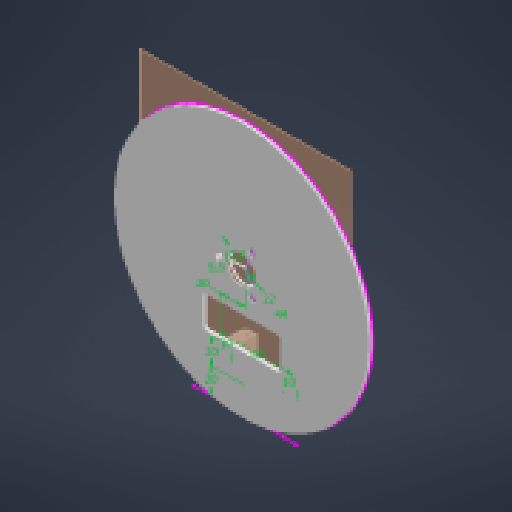
# Autodesk Inventor part: Pokrywa_góra
Saved by Autodesk Inventor 2025 (Build 290162000, 162)
## iProperties
Created: 2024-04-14
Part Number: Pokrywa_góra
Material: Generic
Document SubType Name: Modeling
Designer: sicia
Density: 1 g/cm^3
Appearance: Default
Author: sicia
Autodesk Inventor part; units mm, degrees
ref_plane "YZ Plane" through (0, 0, 0) normal (1, 0, 0) x (0, 1, 0)
ref_plane "XZ Plane" through (0, 0, 0) normal (0, 1, 0) x (-1, 0, 0)
ref_plane "XY Plane" through (0, 0, 0) normal (0, 0, 1) x (1, 0, 0)
ref_plane "Work Plane1" through (0, 0, 0) normal (0, 0, 1) x (1, 0, 0)
ref_plane "Work Plane2" through (0, 0, 0) normal (0, 0, 1) x (1, 0, 0)
sketch "Sketch3" plane through (0, 0, 0) normal (0, 0, 1) x (1, 0, 0)
  circle A0 centre (-75, -25) radius 100 projected
  circle A1 centre (-75, -25) radius 95 projected
  point P0 (-75, -25)
  point P1 (-75, -25)
  point P2 (-75, -25)
  point P3 (-75, -25)
extrude "Extrusion3" add sketch "Sketch3" along normal blind 3 contours A0 | A1
sketch "Sketch9" plane through (0, 0, 0) normal (0, 0, -1) x (-1, 0, 0)
  line L0 (115, -125) -> (35, -125) projected
  line L1 (35, -105) -> (95, -105)
  line L2 (95, -105) -> (95, -85)
  line L3 (95, -85) -> (35, -85)
  line L4 (35, -85) -> (35, -105)
  line L5 (35, -105) -> (95, -85) construction
  line L6 (95, -105) -> (35, -85) construction
  arc A0 (120.4545, -114.0724) -> (120.4545, 64.0724) centre (75, -25) ccw projected
  line L7 (85, -85) -> (85, -105)
  line L8 (45, -85) -> (45, -105)
  point P0 (0, 0)
  point P1 (105.3097, -125)
  point P2 (44.6903, -125)
  point P3 (65, -95)
  point P4 (111.3636, 68.1541)
  point P5 (111.3636, -118.1541)
  point P6 (95, -95)
  point P7 (85, -95)
  point P8 (35, -95)
  point P9 (45, -95)
  dimension "d48" = 60
  dimension "d49" = 20
  dimension "d53" = 10
  dimension "d54" = 10
  dimension "d56" = 20
  dimension "d57" = 20
  constraints: 16 end point, 6 midpoint, 4 point on line, 3 perpendicular, 2 parallel, 1 horizontal
  measures "d48" distance of L3.end L2.end
  measures "d49" distance of L2.end L1.end
  measures "d53" distance of point (95, -95) point (85, -95)
  measures "d54" distance of point (35, -95) point (45, -95)
  measures "d56" distance between parallel lines of L0 L1
  measures "d57" distance from line of A0.centre L2
extrude "Extrusion10" add sketch "Sketch9" along normal blind 20 contours L4 L3 L8 L1 | L7 L3 L2 L1
sketch "Sketch11" plane through (-45, -85, 0) normal (0, 1, 0) x (1, 0, 0)
  circle A0 centre (3.6, 4.915) radius 1.5
  line L0 (0, 20) -> (10, 20) projected
  line L1 (0, 0) -> (0, 20) projected
  circle A1 centre (-43.6, 4.915) radius 1.5
  line L2 (-50, 20) -> (-40, 20) projected
  line L3 (-40, 0) -> (-40, 20) projected
  line L4 (10, 0) -> (-70, 0) projected
  circle A2 centre (3.6, 15.085) radius 1.4068
  circle A3 centre (-43.6, 15.085) radius 1.5
  point P0 (45, 0)
  point P1 (5, 20)
  point P2 (0.3097, 0)
  point P3 (-60.3097, 0)
  dimension "d58" = 3
  dimension "d60" = 3.6
  dimension "d61" = 3
  dimension "d63" = 3.6
  dimension "d66" = 4.915
  dimension "d67" = 4.915
  dimension "d91" = 10.17
  dimension "d92" = 3
  dimension "d94" = 10.17
  constraints: 4 centre point, 1 midpoint
  measures "d58" diameter of A0
  measures "d60" distance from line of L1 A0.centre
  measures "d61" diameter of A1
  measures "d63" distance from line of L3 A1.centre
  measures "d66" distance from line of L4 A1.centre
  measures "d67" distance from line of L4 A0.centre
  measures "d91" distance of A2.centre A0.centre
  measures "d92" diameter of A3
  measures "d94" distance of A1.centre A3.centre
extrude "Extrusion12" cut sketch "Sketch11" against normal blind 20
sketch "Sketch12" plane through (0, 0, 0) normal (0, 0, -1) x (-1, 0, 0)
  line L0 (35, -105) -> (35, -85) projected
  line L1 (35, -85) -> (45, -85) projected
  line L2 (45, -85) -> (45, -105) projected
  line L3 (45, -105) -> (35, -105) projected
  line L4 (95, -85) -> (95, -105) projected
  line L5 (95, -105) -> (85, -105) projected
  line L6 (85, -105) -> (85, -85) projected
  line L7 (85, -85) -> (95, -85) projected
  circle A0 centre (75, -25) radius 11
  circle A1 centre (75, -25) radius 22
  circle A2 centre (75, -25) radius 100 projected
  line L8 (75, -25) -> (92.5, -25)
  circle A3 centre (92.5, -25) radius 2.75
  line L9 (75, -25) -> (66.25, -9.8446)
  circle A4 centre (66.25, -9.8446) radius 2.75
  line L10 (75, -25) -> (66.25, -40.1554)
  circle A5 centre (66.25, -40.1554) radius 2.75
  point P0 (0, 0)
  point P1 (38.6364, 68.1541)
  point P2 (38.6364, -118.1541)
  dimension "d70" = 22
  dimension "d71" = 44
  dimension "d76" = 17.5
  dimension "d77" = 5.5
  constraints: 6 end point, 5 centre point, 3 coincident, 2 concentric, 1 horizontal
  measures "d70" diameter of A0
  measures "d71" diameter of A1
  measures "d76" distance of L8.start L8.end
  measures "d77" diameter of A3
extrude "Extrusion13" cut sketch "Sketch12" against normal blind 35 contours L8 L9 A0 | A0 L10 L8 | L9 L10 A0
extrude "Extrusion14" cut sketch "Sketch12" against normal blind 2 contours A5 | A4 | A3 | A1
extrude "Extrusion15" cut sketch "Sketch12" against normal blind 3 contours A5 | A4 | A3
sketch "Sketch13" plane through (0, 0, 0) normal (0, 0, -1) x (-1, 0, 0)
  point P0 (0, 0)
sketch "Sketch14" plane through (0, 0, 0) normal (0, 0, -1) x (-1, 0, 0)
  line L0 (47, -80) -> (103, -80)
  line L1 (105, -78) -> (105, -57)
  line L2 (103, -55) -> (47, -55)
  line L3 (45, -57) -> (45, -78)
  line L4 (115, -125) -> (35, -125) projected
  circle A0 centre (75, -25) radius 11 projected
  arc A1 (47, -55) -> (45, -57) centre (47, -57) ccw
  arc A2 (103, -80) -> (105, -78) centre (103, -78) ccw
  arc A3 (47, -55) -> (45, -57) centre (47, -57) ccw
  arc A4 (45, -78) -> (47, -80) centre (47, -78) ccw
  arc A5 (105, -57) -> (103, -55) centre (103, -57) ccw
  point P0 (0, 0)
  point P1 (105, -55)
  point P2 (105, -80)
  point P3 (45, -55)
  point P4 (105.3097, -125)
  point P5 (44.6903, -125)
  dimension "d84" = 60
  dimension "d85" = 25
  dimension "d86" = 45
  dimension "d87" = 30
  dimension "d88" = 2
  constraints: 10 point on circle, 10 tangent, 8 end point, 8 point on line, 5 centre point, 4 equal radius, 2 parallel, 1 horizontal, 1 perpendicular
  measures "d84" distance of point (45, -55) point (105, -55)
  measures "d85" distance of point (105, -55) point (105, -80)
  measures "d86" distance between parallel lines of L4 L0
  measures "d87" distance from line of A0.centre L1
  measures "d88" radius of A1
extrude "Extrusion16" cut sketch "Sketch14" against normal blind 20 contours A4 L3 A1 L2 A5 L1 A2 L0
fillet "Fillet1" radius 5 4 edges at (-35, -95, -20) (-35, -95, 0) (-95, -95, 0) (-95, -95, -20)
body "Solid2"
